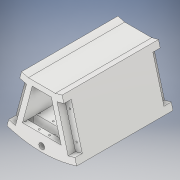
# Autodesk Inventor part: SA001b
Saved by Autodesk Inventor 2017 SP1 (Build 210196100, 196)
## iProperties
Created: 2017-06-04
Part Number: SA001b
Material: ABS Plastic
Document SubType Name: Modeling
Designer: Zach
Density: 1.06 g/cm^3
Appearance: CR White
Author: Zach
Autodesk Inventor part; units mm, degrees
ref_plane "YZ Plane" through (0, 0, 0) normal (1, 0, 0) x (0, 1, 0)
ref_plane "XZ Plane" through (0, 0, 0) normal (0, 1, 0) x (-1, 0, 0)
ref_plane "XY Plane" through (0, 0, 0) normal (0, 0, 1) x (1, 0, 0)
sketch "Sketch1" plane through (0, 0, 0) normal (0, 0, 1) x (1, 0, 0)
  line L0 (0, 0) -> (160, 0)
  line L1 (160, 0) -> (118.589, 154.5481)
  line L2 (41.411, 154.5481) -> (0, 0)
  line L3 (41.411, 154.5481) -> (118.589, 154.5481)
  dimension "d0" = 160
  dimension "d1" = 160
  dimension "d2" = 75
  dimension "d8" = 75
  constraints: 8 end point, 2 horizontal
  measures "d0" distance of L0.start L0.end
  measures "d1" distance of L1.end L0.end
  measures "d2" angle of L1 L0
  measures "d8" angle of L0 L2
extrude "Extrusion1" add sketch "Sketch1" along normal blind 55
sketch "Sketch6" plane through (0, 0, 55) normal (0, 0, 1) x (1, 0, 0)
  line L0 (0, 0) -> (160, 0) construction
  line L1 (160, 0) -> (118.589, 154.5481) construction
  line L2 (118.589, 154.5481) -> (41.411, 154.5481) construction
  line L3 (41.411, 154.5481) -> (0, 0) construction
  line L4 (0, 0) -> (160, 0) construction
  line L5 (19.5484, 15) -> (140.4516, 15) construction
  line L6 (140.4516, 15) -> (107.079, 139.5481) construction
  line L7 (107.079, 139.5481) -> (52.921, 139.5481)
  line L8 (52.921, 139.5481) -> (19.5484, 15) construction
  line L9 (24.9074, 35) -> (135.0926, 35)
  line L10 (107.079, 139.5481) -> (135.0926, 35)
  line L11 (52.921, 139.5481) -> (24.9074, 35)
  dimension "d157" = 15
  dimension "d158" = 35
  constraints: 14 end point, 2 collinear, 2 point on line, 1 horizontal, 3 other
  measures "d157" distance between parallel lines of L3 L8
  measures "d158" distance between parallel lines of L0 L9
extrude "Extrusion5" cut sketch "Sketch6" against normal through all
sketch "Sketch7" plane through (0, 0, 0) normal (0, 0, -1) x (-1, 0, 0)
  circle A0 centre (-80, 304.672) radius 315 construction
  line L0 (0, 0) -> (-160, 0) projected
  arc A1 (-160, 0) -> (0, 0) centre (-80, 304.672) ccw
  dimension "d28" = 630
  constraints: 4 point on circle, 2 centre point, 1 concentric
  measures "d28" diameter of A0
extrude "Extrusion6" add sketch "Sketch7" against normal blind 55
sketch "Sketch21" plane through (24.9074, 35, 55) normal (0, 1, 0) x (1, 0, 0)
  line L0 (135.0926, 55) -> (-24.9074, 55) projected
  line L1 (135.0926, 55) -> (135.0926, 0) projected
  line L2 (-24.9074, 0) -> (135.0926, 0) projected
  line L3 (-24.9074, 55) -> (-24.9074, 0) projected
  line L4 (120.0926, 15) -> (120.0926, 40)
  line L5 (120.0926, 40) -> (-9.9074, 40)
  line L6 (-9.9074, 40) -> (-9.9074, 15)
  line L7 (-9.9074, 15) -> (120.0926, 15)
  point P0 (-85, 55)
  dimension "d159" = 15
  constraints: 8 end point, 3 other
  measures "d159" distance between parallel lines of L2 L7
extrude "Extrusion22" cut sketch "Sketch21" against normal through all contours L7 L6 L5 L4
sketch "Sketch22" plane through (0, 0, 0) normal (0, 0, -1) x (-1, 0, 0)
  line L0 (-41.411, 154.5481) -> (0, 0) projected
  line L1 (-118.589, 154.5481) -> (-41.411, 154.5481) projected
  line L2 (-160, 0) -> (-118.589, 154.5481) projected
  arc A0 (-160, 0) -> (0, 0) centre (-80, 304.672) ccw projected
  line L3 (-52.921, 139.5481) -> (-24.9074, 35) projected
  line L4 (-24.9074, 35) -> (-135.0926, 35) projected
  line L5 (-135.0926, 35) -> (-107.079, 139.5481) projected
  line L6 (-107.079, 139.5481) -> (-52.921, 139.5481) projected
  line L7 (-41.411, 154.5481) -> (0, 0) projected
  line L8 (-118.589, 154.5481) -> (-41.411, 154.5481) projected
  line L9 (-160, 0) -> (-118.589, 154.5481) projected
  arc A1 (-160, 0) -> (0, 0) centre (-80, 304.672) ccw projected
extrude "Extrusion23" add sketch "Sketch22" along normal blind 220
sketch "Sketch24" plane through (24.9074, 35, 15) normal (0, 1, 0) x (1, 0, 0)
  line L0 (109.7368, 7.5) -> (69.7368, 7.5) construction
  line L1 (69.7368, 7.5) -> (69.7368, -32.5) construction
  line L2 (69.7368, -32.5) -> (109.7368, -32.5) construction
  line L3 (109.7368, -32.5) -> (109.7368, 7.5) construction
  line L4 (40.4485, 7.5) -> (0.4485, 7.5) construction
  line L5 (0.4485, 7.5) -> (0.4485, -32.5) construction
  line L6 (0.4485, -32.5) -> (40.4485, -32.5) construction
  line L7 (40.4485, -32.5) -> (40.4485, 7.5) construction
  line L8 (69.7368, -12.5) -> (40.4485, -12.5) construction
  circle A0 centre (109.7368, -32.5) radius 2.5
  circle A1 centre (109.7368, 7.5) radius 2.5
  circle A2 centre (69.7368, 7.5) radius 2.5
  circle A3 centre (69.7368, -32.5) radius 2.5
  circle A4 centre (0.4485, -32.5) radius 2.5
  circle A5 centre (0.4485, 7.5) radius 2.5
  circle A6 centre (40.4485, 7.5) radius 2.5
  circle A7 centre (40.4485, -32.5) radius 2.5
  line L9 (-24.9074, -40) -> (135.0926, -40) projected
  point P0 (-26.0645, 55)
  point P1 (55.0926, -12.5)
  point P2 (55.0926, -40)
  dimension "d141" = 40
  dimension "d142" = 40
  dimension "d143" = 40
  dimension "d144" = 40
  dimension "d145" = 29.2883
  dimension "d147" = 5
  dimension "d148" = 5
  dimension "d149" = 5
  dimension "d150" = 5
  dimension "d151" = 5
  dimension "d152" = 5
  dimension "d153" = 5
  dimension "d154" = 5
  dimension "d160" = 7.5
  constraints: 18 end point, 8 centre point, 8 coincident, 4 midpoint, 4 parallel, 2 horizontal, 2 perpendicular, 1 point on line, 1 vertical alignment
  measures "d141" distance of L2.end L1.end
  measures "d142" distance of L1.end L0.end
  measures "d143" distance of L6.end L5.end
  measures "d144" distance of L5.end L4.end
  measures "d145" distance between parallel lines of L7 L1
  measures "d147" diameter of A0
  measures "d148" diameter of A1
  measures "d149" diameter of A2
  measures "d150" diameter of A3
  measures "d151" diameter of A4
  measures "d152" diameter of A5
  measures "d153" diameter of A6
  measures "d154" diameter of A7
  measures "d160" distance between parallel lines of L9 L2
extrude "Extrusion25" cut sketch "Sketch24" against normal through all
sketch "Sketch25" plane through (0, 0, -220) normal (0, 0, -1) x (-1, 0, 0)
  circle A0 centre (-80, 4.836) radius 8.25
  line L0 (-41.411, 154.5481) -> (-118.589, 154.5481) projected
  point P0 (0, 0)
  point P1 (-80, 154.5481)
  dimension "d161" = 16.5
  dimension "d162" = 149.7122
  constraints: 1 centre point, 1 midpoint, 1 vertical alignment
  measures "d161" diameter of A0
  measures "d162" distance from line of A0.centre L0
extrude "Extrusion26" cut sketch "Sketch25" against normal through all
sketch "Sketch26" plane through (0, 0, -220) normal (0, 0, -1) x (-1, 0, 0)
  line L0 (-107.079, 139.5481) -> (-52.921, 139.5481) projected
  line L1 (-135.0926, 35) -> (-107.079, 139.5481) projected
  line L2 (-24.9074, 35) -> (-135.0926, 35) projected
  line L3 (-52.921, 139.5481) -> (-24.9074, 35) projected
  point P0 (0, 0)
extrude "Extrusion27" add sketch "Sketch26" against normal blind 5
sketch "Sketch27" plane through (0, 0, -220) normal (0, 0, -1) x (-1, 0, 0)
  line L0 (-41.411, 154.5481) -> (-118.589, 154.5481) projected
  line L1 (-118.589, 154.5481) -> (-160, 0) projected
  circle A0 centre (-80, 60) radius 2.5
  circle A1 centre (-71.5, 60) radius 2
  circle A2 centre (-88.5, 60) radius 2
  line L2 (-88.5, 60) -> (-71.5, 60) construction
  point P0 (0, 0)
  point P1 (-80, 154.5481)
  dimension "d167" = 5
  dimension "d168" = 4
  dimension "d169" = 4
  dimension "d170" = 17
  dimension "d188" = 94.5481
  constraints: 3 centre point, 2 end point, 2 midpoint, 1 coincident, 1 horizontal, 1 vertical alignment
  measures "d167" diameter of A0
  measures "d168" diameter of A1
  measures "d169" diameter of A2
  measures "d170" distance of L2.start L2.end
  measures "d188" distance from line of L0 A0.centre
extrude "Extrusion28" cut sketch "Sketch27" against normal through all
sketch "Sketch29" plane through (0, 0, -215) normal (0, 0, 1) x (1, 0, 0)
  circle A0 centre (80, 60) radius 2.5 construction
  circle A1 centre (80, 60) radius 2.5 construction
  circle A2 centre (80, 60) radius 13
  circle A3 centre (80, 60) radius 18
  point P0 (0, 0)
  dimension "d177" = 26
  dimension "d178" = 5
  constraints: 2 centre point, 1 coincident
  measures "d177" diameter of A2
  measures "d178" radial gap between concentric circles of A2 A3
extrude "Extrusion30" add sketch "Sketch29" along normal blind 25
sketch "Sketch31" plane through (80, 60, -215) normal (0, 0, 1) x (1, 0, 0)
  circle A0 centre (0, 0) radius 2.5 projected
  circle A1 centre (0, 0) radius 3.5
  point P0 (-80, -60)
  dimension "d181" = 7
  constraints: 1 centre point, 1 coincident
  measures "d181" diameter of A1
extrude "Extrusion31" cut sketch "Sketch31" against normal blind 3
sketch "Sketch32" plane through (0, 0, -220) normal (0, 0, -1) x (-1, 0, 0)
  circle A0 centre (-88.5, 60) radius 2 projected
  circle A1 centre (-71.5, 60) radius 2 projected
  circle A2 centre (-88.5, 60) radius 4
  circle A3 centre (-71.5, 60) radius 2 projected
  circle A4 centre (-71.5, 60) radius 4
  point P0 (0, 0)
  dimension "d184" = 8
  dimension "d185" = 8
  constraints: 2 centre point, 2 coincident
  measures "d184" diameter of A2
  measures "d185" diameter of A4
extrude "Extrusion32" cut sketch "Sketch32" against normal blind 3
sketch "Sketch33" plane through (118.589, 154.5481, 55) normal (0.9659258, 0.258819, 0) x (0, 0, -1)
  line L0 (275, 0) -> (0, 0) projected
  line L1 (0, -160) -> (0, 0) projected
  line L2 (275, -160) -> (0, -160) projected
  line L3 (275, 0) -> (275, -160) projected
  point P0 (55, -118.589)
extrude "Extrusion33" add sketch "Sketch33" along normal blind 20
sketch "Sketch34" plane through (0, 0, -220) normal (-0.9659258, 0.258819, 0) x (0, 0, 1)
  line L0 (0, 0) -> (275, 0) projected
  line L1 (275, 160) -> (275, 0) projected
  line L2 (0, 160) -> (275, 160) projected
  line L3 (0, 0) -> (0, 160) projected
  point P0 (220, 0)
extrude "Extrusion34" add sketch "Sketch34" along normal blind 20
sketch "Sketch35" plane through (0, 0, -220) normal (0, 0, -1) x (-1, 0, 0)
  line L0 (0, 0) -> (19.3185, 5.1764) construction
  line L1 (-22.0925, 159.7245) -> (19.3185, 5.1764) construction
  line L2 (-41.411, 154.5481) -> (-22.0925, 159.7245) construction
  line L3 (-118.589, 154.5481) -> (-137.9075, 159.7245) construction
  line L4 (-179.3185, 5.1764) -> (-137.9075, 159.7245) construction
  line L5 (-160, 0) -> (-179.3185, 5.1764) construction
  line L6 (-41.411, 154.5481) -> (-118.589, 154.5481) construction
  line L7 (0, 0) -> (-41.411, 154.5481) construction
  arc A0 (-160, 0) -> (0, 0) centre (-80, 304.672) ccw construction
  line L8 (-160, 0) -> (-118.589, 154.5481) construction
  line L9 (14.401, 23.529) -> (-4.9176, 18.3526)
  line L10 (-36.4935, 136.1955) -> (-17.175, 141.3719)
  line L11 (-123.5065, 136.1955) -> (-142.825, 141.3719)
  line L12 (-155.0824, 18.3526) -> (-174.401, 23.529)
  line L13 (-4.9176, 18.3526) -> (-36.4935, 136.1955)
  line L14 (-17.175, 141.3719) -> (14.401, 23.529)
  line L15 (19.3185, 5.1764) -> (-22.0925, 159.7245) projected
  line L16 (-155.0824, 18.3526) -> (-123.5065, 136.1955)
  line L17 (-142.825, 141.3719) -> (-174.401, 23.529)
  dimension "d202" = 19
  dimension "d203" = 19
  dimension "d204" = 19
  dimension "d205" = 19
  constraints: 20 end point, 8 point on line, 4 perpendicular, 2 collinear, 1 parallel
  measures "d202" distance between parallel lines of L0 L9
  measures "d203" distance between parallel lines of L2 L10
  measures "d204" distance between parallel lines of L3 L11
  measures "d205" distance between parallel lines of L5 L12
extrude "Extrusion35" cut sketch "Sketch35" against normal blind 21
sketch "Sketch36" plane through (0, 0, -199) normal (0, 0, -1) x (-1, 0, 0)
  line L0 (-142.825, 141.3719) -> (-123.5065, 136.1955) construction
  line L1 (-174.401, 23.529) -> (-142.825, 141.3719) construction
  line L2 (-155.0824, 18.3526) -> (-174.401, 23.529) construction
  line L3 (-123.5065, 136.1955) -> (-155.0824, 18.3526) construction
  line L4 (14.401, 23.529) -> (-4.9176, 18.3526) construction
  line L5 (-17.175, 141.3719) -> (14.401, 23.529) construction
  line L6 (-36.4935, 136.1955) -> (-17.175, 141.3719) construction
  line L7 (-4.9176, 18.3526) -> (-36.4935, 136.1955) construction
  circle A0 centre (-139.248, 116.0845) radius 2.5
  line L8 (-139.2945, 77.2741) -> (-158.613, 82.4504) construction
  line L9 (-20.7055, 77.2741) -> (-1.387, 82.4504) construction
  line L10 (-139.248, 116.0845) -> (-158.6594, 43.64) construction
  circle A1 centre (-158.6594, 43.64) radius 2.5
  line L11 (-20.752, 116.0845) -> (-1.3406, 43.64) construction
  circle A2 centre (-1.3406, 43.64) radius 2.5
  circle A3 centre (-20.752, 116.0845) radius 2.5
  point P0 (-148.9537, 79.8623)
  point P1 (-11.0463, 79.8623)
  dimension "d206" = 5
  dimension "d210" = 5
  dimension "d211" = 75
  dimension "d212" = 5
  dimension "d213" = 5
  dimension "d214" = 75
  constraints: 8 end point, 8 midpoint, 4 centre point, 4 coincident, 2 perpendicular, 1 parallel
  measures "d206" diameter of A0
  measures "d210" diameter of A1
  measures "d211" distance of L10.start L10.end
  measures "d212" diameter of A2
  measures "d213" diameter of A3
  measures "d214" distance of L11.start L11.end
extrude "Extrusion36" cut sketch "Sketch36" against normal through all
sketch "Sketch38" plane through (0, 0, 55) normal (0, 0, 1) x (1, 0, 0)
  line L0 (123.5065, 136.1955) -> (155.0824, 18.3526) projected
  line L1 (174.401, 23.529) -> (142.825, 141.3719) projected
  line L2 (142.825, 141.3719) -> (123.5065, 136.1955) projected
  line L3 (174.401, 23.529) -> (142.825, 141.3719) projected
  line L4 (155.0824, 18.3526) -> (174.401, 23.529) projected
  line L5 (123.5065, 136.1955) -> (155.0824, 18.3526) projected
  line L6 (-14.401, 23.529) -> (4.9176, 18.3526) projected
  line L7 (17.175, 141.3719) -> (-14.401, 23.529) projected
  line L8 (36.4935, 136.1955) -> (17.175, 141.3719) projected
  line L9 (4.9176, 18.3526) -> (36.4935, 136.1955) projected
  point P0 (0, 0)
extrude "Extrusion38" cut sketch "Sketch38" against normal blind 21
body "Solid1"
